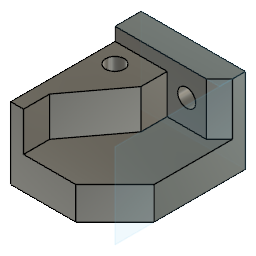
Test_piece1 robocon v1 (Autodesk Fusion 360 design; units mm, degrees)
Autodesk Fusion 360 part; units mm, degrees
sketch "Sketch1" plane through (0, 0, 0) normal (0, 0, 1) x (1, 0, 0)
  line L0 (8, 10) -> (-8, 10)
  line L1 (-8, 10) -> (-8, -10)
  line L2 (-8, -10) -> (8, -10)
  line L3 (8, -10) -> (8, 10)
  line L4 (8, 10) -> (-8, -10) construction
  line L5 (-8, 10) -> (8, -10) construction
  dimension "d1" = 16
  dimension "d2" = 20
  constraint horizontal L0
  constraint perpendicular L0 L1
  constraint parallel L0 L2
  constraint parallel L1 L3
  constraint coincident L4 origin
  constraint coincident L5 origin
  measures "d1" distance of L1.end L2.end
  measures "d2" distance of L0.end L1.end
extrude "Extrude1" add sketch "Sketch1" along normal blind 13
sketch "Sketch2" plane through (8, 0, 0) normal (1, 0, 0) x (0, 1, 0)
  line L0 (-10, 0) -> (10, 0)
  line L1 (10, 0) -> (10, 13)
  line L2 (10, 13) -> (-10, 13)
  line L3 (-10, 13) -> (-10, 0)
sketch "Sketch3" plane through (0, 10, 0) normal (0, 1, 0) x (-1, 0, 0)
  line L0 (-8, 0) -> (8, 0)
  line L1 (8, 0) -> (8, 13)
  line L2 (8, 13) -> (-8, 13)
  line L3 (-8, 13) -> (-8, 0)
sketch "Sketch4" plane through (0, 0, 13) normal (0, 0, 1) x (-1, 0, 0)
  line L0 (-8, 10) -> (-8, -10)
  line L1 (-8, -10) -> (8, -10)
  line L2 (8, -10) -> (8, 10)
  line L3 (8, 10) -> (-8, 10)
  line L4 (8, -6) -> (-8, -6)
  line L5 (-8, -6) -> (-8, 10)
  line L6 (-8, 10) -> (8, 10)
  line L7 (8, 10) -> (8, -6)
  line L8 (8, -6) -> (-8, 10) construction
  line L9 (-8, -6) -> (8, 10) construction
  point P0 (0, 2)
  dimension "d5" = 16
  dimension "d6" = 16
  constraint horizontal L4
  constraint perpendicular L4 L5
  constraint parallel L4 L6
  constraint parallel L5 L7
  constraint coincident L8 P0
  constraint coincident L9 P0
  measures "d5" distance of L0.start L2.end
  measures "d6" distance of L4.end L0.start
extrude "Extrude2" cut sketch "Sketch4" against normal blind 2 contours L0 L2 L3 L4 L5 L6 L7
sketch "Sketch5" plane through (0, 0, 11) normal (0, 0, 1) x (-1, 0, 0)
  line L0 (8, 10) -> (-8, 10)
  line L1 (-8, 10) -> (-8, -6)
  line L2 (-8, -6) -> (8, -6)
  line L3 (8, -6) -> (8, 10)
  line L4 (0, -6) -> (-8, -6)
  line L5 (-8, -6) -> (-8, 10)
  line L6 (-8, 10) -> (0, 10)
  line L7 (0, 10) -> (0, -6)
  line L8 (0, -6) -> (-8, 10) construction
  line L9 (-8, -6) -> (0, 10) construction
  point P0 (-4, 2)
  dimension "d9" = 8
  dimension "d10" = 16
  constraint horizontal L4
  constraint perpendicular L4 L5
  constraint parallel L4 L6
  constraint parallel L5 L7
  constraint coincident L8 P0
  constraint coincident L9 P0
  measures "d9" distance of L0.end L6.end
  measures "d10" distance of L1.end L0.end
extrude "Extrude3" cut sketch "Sketch5" against normal blind 6 contours L0 L1 L2 L4 L5 L6 L7
sketch "Sketch6" plane through (0, 0, 11) normal (0, 0, 1) x (-1, 0, 0)
  line L0 (0, 10) -> (0, -6)
  line L1 (0, -6) -> (8, -6)
  line L2 (8, -6) -> (8, 10)
  line L3 (8, 10) -> (0, 10)
  line L4 (6, 6) -> (0, 6)
  line L5 (0, 6) -> (0, 10)
  line L6 (0, 10) -> (6, 10)
  line L7 (6, 10) -> (6, 6)
  line L8 (6, 6) -> (0, 10) construction
  line L9 (0, 6) -> (6, 10) construction
  point P0 (3, 8)
  dimension "d13" = 6
  dimension "d14" = 4
  constraint horizontal L4
  constraint perpendicular L4 L5
  constraint parallel L4 L6
  constraint parallel L5 L7
  constraint coincident L8 P0
  constraint coincident L9 P0
  measures "d13" distance of L0.start L6.end
  measures "d14" distance of L4.end L0.start
extrude "Extrude4" cut sketch "Sketch6" against normal blind 6 contours L0 L3 L4 L5 L6 L7
sketch "Sketch7" plane through (0, 0, 11) normal (0, 0, 1) x (-1, 0, 0)
  line L0 (6, 6) -> (0, 6)
  line L1 (0, 6) -> (0, -6)
  line L2 (0, -6) -> (8, -6)
  line L3 (8, -6) -> (8, 10)
  line L4 (8, 10) -> (6, 10)
  line L5 (6, 10) -> (6, 6)
  line L6 (6, 6) -> (0, -1.9864)
  line L7 (0, 6) -> (0, -1.9864)
  constraint coincident L0.start L5.end
  constraint coincident L1 L6.end
  constraint coincident L0.end L1.start
extrude "Extrude5" cut sketch "Sketch7" against normal blind 6 contours L0 L1 L6 L7
sketch "Sketch8" plane through (0, 0, 13) normal (0, 0, 1) x (-1, 0, 0)
  line L0 (8, -6) -> (-8, -6)
  line L1 (-8, -6) -> (-8, -10)
  line L2 (-8, -10) -> (8, -10)
  line L3 (8, -10) -> (8, -6)
sketch "Sketch9" plane through (0, 0, 13) normal (0, 0, 1) x (1, 0, 0)
  line L0 (6, 6) -> (8, 8)
  line L1 (8, 8) -> (8, 6)
  line L2 (8, 6) -> (6, 6)
  constraint vertical L1
  constraint perpendicular L1 L2
extrude "Extrude6" cut sketch "Sketch9" against normal blind 8
chamfer "Chamfer1" distance 6 angle 45 1 edges at (8, -10, 2.5)
sketch "Sketch10" plane through (0, 6, 0) normal (0, -1, 0) x (1, 0, 0)
  line L0 (6, 5) -> (6, 13)
  line L1 (6, 13) -> (-8, 13)
  line L2 (-8, 13) -> (-8, 11)
  line L3 (-8, 11) -> (0, 11)
  line L4 (0, 11) -> (0, 5)
  line L5 (0, 5) -> (6, 5)
  circle A0 centre (2.9897, 9) radius 1.3799
extrude "Extrude7" cut sketch "Sketch10" against normal blind 4 contours A0
sketch "Sketch11" plane through (0, 0, 11) normal (0, 0, 1) x (-1, 0, 0)
  line L0 (6, 6) -> (0, -1.9864)
  line L1 (0, -1.9864) -> (0, -6)
  line L2 (0, -6) -> (8, -6)
  line L3 (8, -6) -> (8, 10)
  line L4 (8, 10) -> (6, 10)
  line L5 (6, 10) -> (6, 6)
  circle A0 centre (5, -3) radius 1.4142
extrude "Extrude8" cut sketch "Sketch11" against normal blind 11 contours A0
